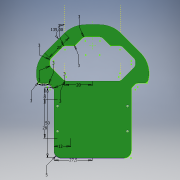
# Autodesk Inventor part: mainpcb
Saved by Autodesk Inventor 2016 (Build 200138000, 138)
## iProperties
Created: 2017-05-27
Part Number: mainpcb
Material: Ogólny
Document SubType Name: Modeling
Designer: Karol
Density: 1 g/cm^3
Appearance: Smooth - Dark Forest Green
Author: Karol
Autodesk Inventor part; units mm, degrees
ref_plane "YZ Plane" through (0, 0, 0) normal (1, 0, 0) x (0, 1, 0)
ref_plane "XZ Plane" through (0, 0, 0) normal (0, 1, 0) x (-1, 0, 0)
ref_plane "XY Plane" through (0, 0, 0) normal (0, 0, 1) x (1, 0, 0)
sketch "Sketch1" plane through (0, 0, 0) normal (0, 1, 0) x (-1, 0, 0)
  line L0 (0, 0) -> (0, 22.5)
  line L1 (5, 27.5) -> (48.7574, 27.5)
  arc A0 (5, 27.5) -> (0, 22.5) centre (5, 22.5) ccw
  arc A1 (95.1955, 5) -> (89.1353, 20) centre (73.6017, 5) ccw
  line L2 (89.1353, 20) -> (74.9931, 34.1421)
  line L3 (89.1353, 20) -> (109.1353, 20) construction
  line L4 (26, 0) -> (39.959, 0)
  line L5 (95.1955, 5) -> (95.1955, 0)
  line L6 (0, 0) -> (0, -22.5)
  arc A2 (0, -22.5) -> (5, -27.5) centre (5, -22.5) ccw
  line L7 (89.1353, 20) -> (109.1353, 20) construction
  line L8 (50.8787, 28.3787) -> (52.6569, 30.1569)
  line L9 (54.8259, 20.1488) -> (64.5921, 20.1488) construction
  line L10 (50, 27.5) -> (65, 27.5) construction
  line L11 (54.8259, 20.1488) -> (64.5921, 20.1488) construction
  line L12 (54.8259, 20.1488) -> (67.5921, 20.1488) construction
  line L13 (53.5355, 32.2782) -> (53.5355, 36.7771)
  arc A3 (74.9931, 34.1421) -> (55.8844, 39.7056) centre (60.372, 19.521) ccw
  line L14 (71.3025, 29.8051) -> (79.3826, 21.725)
  line L15 (81.1398, 11.9677) -> (85.7467, 7.3603)
  line L16 (86.6252, 5.2391) -> (86.6252, 0)
  line L17 (54.8259, 0) -> (54.8259, 18.7574)
  line L18 (55.7045, 20.8787) -> (64.6301, 29.805)
  line L19 (66.7515, 30.6838) -> (69.1812, 30.6838)
  line L20 (80.2613, 19.6037) -> (80.2613, 14.0889)
  arc A4 (71.3025, 29.8051) -> (69.1812, 30.6838) centre (69.1812, 27.6838) ccw
  arc A5 (66.7515, 30.6838) -> (64.6301, 29.805) centre (66.7515, 27.6838) ccw
  arc A6 (55.7045, 20.8787) -> (54.8259, 18.7574) centre (57.8259, 18.7574) ccw
  arc A7 (48.7574, 27.5) -> (50.8787, 28.3787) centre (48.7574, 30.5) ccw
  arc A8 (52.6569, 30.1569) -> (53.5355, 32.2782) centre (50.5355, 32.2782) ccw
  arc A9 (55.8844, 39.7056) -> (53.5355, 36.7771) centre (56.5355, 36.7771) ccw
  arc A10 (80.2613, 19.6037) -> (79.3826, 21.725) centre (77.2613, 19.6037) ccw
  arc A11 (80.2613, 14.0889) -> (81.1398, 11.9677) centre (83.2613, 14.0889) ccw
  arc A12 (86.6252, 5.2391) -> (85.7467, 7.3603) centre (83.6252, 5.2391) ccw
  arc A13 (89.1353, -20) -> (95.1955, -5) centre (73.6017, -5) ccw
  line L21 (89.1353, -20) -> (74.9931, -34.1421)
  line L22 (89.1353, -20) -> (109.1353, -20) construction
  line L23 (95.1955, -5) -> (95.1955, 0)
  line L24 (89.1353, -20) -> (109.1353, -20) construction
  line L25 (50.8787, -28.3787) -> (52.6569, -30.1569)
  line L26 (54.8259, -20.1488) -> (64.5921, -20.1488) construction
  line L27 (54.8259, -20.1488) -> (64.5921, -20.1488) construction
  line L28 (54.8259, -20.1488) -> (67.5921, -20.1488) construction
  line L29 (50, -27.5) -> (65, -27.5) construction
  line L30 (53.5355, -32.2782) -> (53.5355, -36.7771)
  arc A14 (55.8844, -39.7056) -> (74.9931, -34.1421) centre (60.372, -19.521) ccw
  line L31 (71.3025, -29.8051) -> (79.3826, -21.725)
  line L32 (81.1398, -11.9677) -> (85.7467, -7.3603)
  line L33 (86.6252, -5.2391) -> (86.6252, 0)
  line L34 (54.8259, 0) -> (54.8259, -18.7574)
  line L35 (55.7045, -20.8787) -> (64.6301, -29.805)
  line L36 (66.7515, -30.6838) -> (69.1812, -30.6838)
  line L37 (80.2613, -19.6037) -> (80.2613, -14.0889)
  arc A15 (69.1812, -30.6838) -> (71.3025, -29.8051) centre (69.1812, -27.6838) ccw
  arc A16 (64.6301, -29.805) -> (66.7515, -30.6838) centre (66.7515, -27.6838) ccw
  arc A17 (54.8259, -18.7574) -> (55.7045, -20.8787) centre (57.8259, -18.7574) ccw
  arc A18 (50.8787, -28.3787) -> (48.7574, -27.5) centre (48.7574, -30.5) ccw
  arc A19 (53.5355, -32.2782) -> (52.6569, -30.1569) centre (50.5355, -32.2782) ccw
  arc A20 (53.5355, -36.7771) -> (55.8844, -39.7056) centre (56.5355, -36.7771) ccw
  arc A21 (79.3826, -21.725) -> (80.2613, -19.6037) centre (77.2613, -19.6037) ccw
  arc A22 (81.1398, -11.9677) -> (80.2613, -14.0889) centre (83.2613, -14.0889) ccw
  arc A23 (85.7467, -7.3603) -> (86.6252, -5.2391) centre (83.6252, -5.2391) ccw
  line L38 (48.7574, -27.5) -> (5, -27.5)
  point P0 (0, 27.5)
  point P1 (80, 0)
  point P2 (42, 25)
  point P3 (14, 25)
  point P4 (14, 15.5)
  point P5 (37, 25)
  point P6 (19, 25)
  point P7 (0, -27.5)
  point P8 (42, -25)
  point P9 (14, -25)
  point P10 (14, -15.5)
  point P11 (37, -25)
  point P12 (19, -25)
  point P13 (80.2613, 20.8464)
  point P14 (53.5355, 31.0355)
  point P15 (53.5355, 39.0355)
  point P16 (70.4238, 30.6838)
  point P17 (80.2613, 12.8464)
  point P18 (86.6252, 6.4816)
  point P19 (54.8259, 20)
  point P20 (65.5088, 30.6838)
  point P21 (80.2613, -20.8464)
  point P22 (53.5355, -31.0355)
  point P23 (53.5355, -39.0355)
  point P24 (70.4238, -30.6838)
  point P25 (80.2613, -12.8464)
  point P26 (86.6252, -6.4816)
  point P27 (54.8259, -20)
  point P28 (65.5088, -30.6838)
  dimension "d2" = 27.5
  dimension "d3" = 50
  dimension "d19" = 5
  dimension "d42" = 8
  dimension "d43" = 28
  dimension "d45" = 12
  dimension "d73" = 20
  dimension "d74" = 135
  dimension "d105" = 5
  dimension "d118" = 8
  dimension "d123" = 20
  dimension "d124" = 3
  dimension "d125" = 3
  dimension "d126" = 3
  dimension "d127" = 3
  dimension "d128" = 3
  dimension "d129" = 3
  dimension "d130" = 3
  dimension "d131" = 3
  dimension "d132" = 3
  constraints: 78 end point, 58 symmetric about line, 50 point on circle, 36 point on line, 24 centre point, 22 tangent, 6 vertical, 5 horizontal, 1 equal length, 12 other
  measures "d2" distance of L0.start point (0, 27.5)
  measures "d3" distance of point (0, 27.5) L10.start
  measures "d19" radius of A0
  measures "d42" horizontal distance of L10.start point (42, 25)
  measures "d43" distance of point (14, 25) point (42, 25)
  measures "d45" distance from line of L1 point (14, 15.5)
  measures "d73" distance of L2.start L2.end
  measures "d74" angle of L3 L2
  measures "d105" distance of L10.start point (53.536, 31.036)
  measures "d118" distance of point (53.536, 31.036) point (53.536, 39.036)
  measures "d123" distance of L17.start point (54.826, 20)
  measures "d124" radius of A4
  measures "d125" radius of A5
  measures "d126" radius of A6
  measures "d127" radius of A7
  measures "d128" radius of A8
  measures "d129" radius of A9
  measures "d130" radius of A10
  measures "d131" radius of A11
  measures "d132" radius of A12
extrude "Extrusion1" add sketch "Sketch1" along normal blind 1.4
hole "Hole1" at (-37, 0, 25) at (-19, 0, 25) at (-37, 0, -25) at (-19, 0, -25) direction (0, 1, 0) diameter 2 depth 2 tip angle 118
hole "Hole3" at (-14, 0, 15.5) direction (0, 1, 0) diameter 0.1 depth 8 tip angle 118
body "Solid1"
